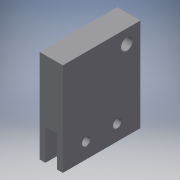
# Autodesk Inventor part: WideSupportForLift
Saved by Autodesk Inventor 2016 SP1 (Build 200210100, 210)
## iProperties
Created: 2016-02-14
Part Number: WideSupportForLift
Material: Aluminum 6061
Document SubType Name: Modeling
Designer: steele
Density: 2.7 g/cm^3
Appearance: Aluminum - Flat
Mass: 201.89 g
Surface Area: 182.87 cm^2
Volume: 74.7739 cm^3
Author: steele
Autodesk Inventor part; units mm, degrees
ref_plane "YZ Plane" through (0, 0, 0) normal (1, 0, 0) x (0, 1, 0)
ref_plane "XZ Plane" through (0, 0, 0) normal (0, 1, 0) x (-1, 0, 0)
ref_plane "XY Plane" through (0, 0, 0) normal (0, 0, 1) x (1, 0, 0)
sketch "Sketch6" plane through (0, 0, 0) normal (1, 0, 0) x (0, 1, 0)
  line L0 (-25.4, 31.75) -> (-25.4, -31.75)
  line L1 (-25.4, -31.75) -> (0, -31.75)
  line L2 (0, -31.75) -> (0, 31.75)
  line L3 (0, 31.75) -> (-25.4, 31.75)
  line L4 (-25.4, 31.75) -> (0, -31.75) construction
  line L5 (-25.4, -31.75) -> (0, 31.75) construction
  line L6 (0, 31.75) -> (0, -31.75)
  line L7 (0, -31.75) -> (50.8, -31.75)
  line L8 (50.8, -31.75) -> (50.8, 31.75)
  line L9 (50.8, 31.75) -> (0, 31.75)
  line L10 (0, 31.75) -> (50.8, -31.75) construction
  line L11 (0, -31.75) -> (50.8, 31.75) construction
  circle A0 centre (39.6875, -20.6375) radius 4.7625
  point P0 (0, 0)
  point P1 (-12.7, 0)
  point P2 (25.4, 0)
  dimension "d12" = 12.7
  dimension "d13" = 25.4
  dimension "d14" = 50.8
  dimension "d15" = 25.4
  dimension "d16" = 9.525
  dimension "d17" = 11.1125
  dimension "d18" = 11.1125
  dimension "d24" = 63.5
  constraints: 24 end point, 6 parallel, 4 midpoint, 2 perpendicular, 1 centre point, 1 vertical
  measures "d12" distance of point (-12.7, 0) point (0, 0)
  measures "d13" distance of point (0, 0) point (25.4, 0)
  measures "d14" distance of L8.end L6.start
  measures "d15" distance of L2.end L0.start
  measures "d16" diameter of A0
  measures "d17" distance from line of A0.centre L7
  measures "d18" distance from line of A0.centre L8
  measures "d24" distance of L0.start L0.end
extrude "Extrusion3" add sketch "Sketch6" along normal mid plane 19.05
sketch "Sketch7" plane through (-9.525, -25.4, 31.75) normal (0, 0, 1) x (1, 0, 0)
  line L0 (9.525, 25.4) -> (9.525, 0) construction
  line L1 (0, 0) -> (19.05, 0) construction
  line L2 (4.7625, 0) -> (14.2875, 0)
  line L3 (14.2875, 0) -> (14.2875, 25.4)
  line L4 (14.2875, 25.4) -> (4.7625, 25.4)
  line L5 (4.7625, 25.4) -> (4.7625, 0)
  line L6 (4.7625, 0) -> (14.2875, 25.4) construction
  line L7 (14.2875, 0) -> (4.7625, 25.4) construction
  point P0 (9.525, 12.7)
  dimension "d21" = 9.525
  constraints: 14 end point, 4 midpoint, 2 parallel, 1 horizontal, 1 perpendicular
  measures "d21" distance between parallel lines of L3 L5
extrude "Extrusion4" cut sketch "Sketch7" against normal through all
sketch "Sketch8" plane through (9.525, 0, 0) normal (1, 0, 0) x (0, 0, -1)
  line L0 (31.75, -25.4) -> (31.75, 0) projected
  line L1 (-31.75, -25.4) -> (31.75, -25.4) projected
  line L2 (-31.75, 0) -> (-31.75, -25.4) projected
  line L3 (-31.75, 0) -> (31.75, 0) projected
  line L4 (-292.1, -85.725) -> (-292.1, -12.7) projected
  arc A0 (-292.1, -85.725) -> (-279.4, -98.425) centre (-279.4, -85.725) ccw projected
  line L5 (222.25, -98.425) -> (-279.4, -98.425) projected
  arc A1 (222.25, -98.425) -> (234.95, -85.725) centre (222.25, -85.725) ccw projected
  line L6 (234.95, -81.1401) -> (234.95, -85.725) projected
  arc A2 (234.95, -81.1401) -> (231.6119, -72.5584) centre (222.25, -81.1401) ccw projected
  line L7 (231.6119, -72.5584) -> (168.8751, -4.1183) projected
  arc A3 (168.8751, -4.1183) -> (159.5132, 0) centre (159.5132, -12.7) ccw projected
  line L8 (159.5132, 0) -> (-279.4, 0) projected
  arc A4 (-279.4, 0) -> (-292.1, -12.7) centre (-279.4, -12.7) ccw projected
  circle A5 centre (215.9, -79.375) radius 4.826 projected
  circle A6 centre (-241.3, -79.375) radius 4.826 projected
  circle A7 centre (200.025, -79.375) radius 4.826 projected
  circle A8 centre (182.9995, -40.6685) radius 3.3782 projected
  circle A9 centre (165.1, -85.725) radius 3.3782 projected
  line L9 (-236.5375, -55.8157) -> (-236.5375, -25.4) projected
  arc A10 (-233.3625, -22.225) -> (-236.5375, -25.4) centre (-233.3625, -25.4) ccw projected
  line L10 (-233.3625, -22.225) -> (-210.2431, -22.225) projected
  arc A11 (-207.7154, -27.3213) -> (-210.2431, -22.225) centre (-210.2431, -25.4) ccw projected
  line L11 (-207.7154, -27.3213) -> (-230.8348, -57.737) projected
  arc A12 (-236.5375, -55.8157) -> (-230.8348, -57.737) centre (-233.3625, -55.8157) ccw projected
  line L12 (-229.0307, -71.1037) -> (-201.0846, -34.338) projected
  arc A13 (-195.3819, -36.2593) -> (-201.0846, -34.338) centre (-198.5569, -36.2593) ccw projected
  line L13 (-195.3819, -36.2593) -> (-195.3819, -73.025) projected
  arc A14 (-198.5569, -76.2) -> (-195.3819, -73.025) centre (-198.5569, -73.025) ccw projected
  line L14 (-198.5569, -76.2) -> (-226.503, -76.2) projected
  arc A15 (-229.0307, -71.1037) -> (-226.503, -76.2) centre (-226.503, -73.025) ccw projected
  line L15 (-73.119, -73.025) -> (-73.119, -34.8804) projected
  arc A16 (-67.6008, -32.738) -> (-73.119, -34.8804) centre (-69.944, -34.8804) ccw projected
  line L16 (-67.6008, -32.738) -> (-32.724, -70.8826) projected
  arc A17 (-35.0672, -76.2) -> (-32.724, -70.8826) centre (-35.0672, -73.025) ccw projected
  line L17 (-35.0672, -76.2) -> (-69.944, -76.2) projected
  arc A18 (-73.119, -73.025) -> (-69.944, -76.2) centre (-69.944, -73.025) ccw projected
  line L18 (34.0449, -27.5424) -> (-2.4193, -67.4233) projected
  arc A19 (-7.9375, -65.2808) -> (-2.4193, -67.4233) centre (-4.7625, -65.2808) ccw projected
  line L19 (-7.9375, -65.2808) -> (-7.9375, -25.4) projected
  arc A20 (-4.7625, -22.225) -> (-7.9375, -25.4) centre (-4.7625, -25.4) ccw projected
  line L20 (-4.7625, -22.225) -> (31.7017, -22.225) projected
  arc A21 (34.0449, -27.5424) -> (31.7017, -22.225) centre (31.7017, -25.4) ccw projected
  line L21 (-22.9807, -67.4233) -> (-59.4449, -27.5424) projected
  arc A22 (-57.1017, -22.225) -> (-59.4449, -27.5424) centre (-57.1017, -25.4) ccw projected
  line L22 (-57.1017, -22.225) -> (-20.6375, -22.225) projected
  arc A23 (-17.4625, -25.4) -> (-20.6375, -22.225) centre (-20.6375, -25.4) ccw projected
  line L23 (-17.4625, -25.4) -> (-17.4625, -65.2808) projected
  arc A24 (-22.9807, -67.4233) -> (-17.4625, -65.2808) centre (-20.6375, -65.2808) ccw projected
  line L24 (47.719, -34.8804) -> (47.719, -73.025) projected
  arc A25 (44.544, -76.2) -> (47.719, -73.025) centre (44.544, -73.025) ccw projected
  line L25 (44.544, -76.2) -> (9.6672, -76.2) projected
  arc A26 (7.324, -70.8826) -> (9.6672, -76.2) centre (9.6672, -73.025) ccw projected
  line L26 (7.324, -70.8826) -> (42.2008, -32.738) projected
  arc A27 (47.719, -34.8804) -> (42.2008, -32.738) centre (44.544, -34.8804) ccw projected
  line L27 (84.1375, -25.4) -> (84.1375, -73.025) projected
  arc A28 (80.9625, -76.2) -> (84.1375, -73.025) centre (80.9625, -73.025) ccw projected
  line L28 (80.9625, -76.2) -> (60.419, -76.2) projected
  arc A29 (57.244, -73.025) -> (60.419, -76.2) centre (60.419, -73.025) ccw projected
  line L29 (57.244, -73.025) -> (57.244, -25.4) projected
  arc A30 (60.419, -22.225) -> (57.244, -25.4) centre (60.419, -25.4) ccw projected
  line L30 (60.419, -22.225) -> (80.9625, -22.225) projected
  arc A31 (84.1375, -25.4) -> (80.9625, -22.225) centre (80.9625, -25.4) ccw projected
  line L31 (142.875, -69.85) -> (142.875, -29.1831) projected
  arc A32 (148.4044, -27.053) -> (142.875, -29.1831) centre (146.05, -29.1831) ccw projected
  line L32 (148.4044, -27.053) -> (188.0708, -70.8949) projected
  arc A33 (185.7165, -76.2) -> (188.0708, -70.8949) centre (185.7165, -73.025) ccw projected
  line L33 (185.7165, -76.2) -> (149.225, -76.2) projected
  arc A34 (142.875, -69.85) -> (149.225, -76.2) centre (149.225, -69.85) ccw projected
  circle A35 centre (-173.7792, -57.6072) radius 5.5626 projected
  circle A36 centre (-96.3092, -32.2072) radius 5.5626 projected
  circle A37 centre (-173.7792, -32.2072) radius 5.5626 projected
  circle A38 centre (-96.3092, -57.6072) radius 5.5626 projected
  circle A39 centre (101.6, -28.575) radius 2.5527 projected
  circle A40 centre (111.125, -19.05) radius 2.5527 projected
  circle A41 centre (120.65, -9.525) radius 2.5527 projected
  circle A42 centre (101.6, -88.9) radius 2.5527 projected
  circle A43 centre (120.65, -69.85) radius 2.5527 projected
  circle A44 centre (111.125, -79.375) radius 2.5527 projected
  circle A45 centre (-266.7, -12.7) radius 3.3782 projected
  circle A46 centre (-266.7, -85.725) radius 3.3782 projected
  circle A47 centre (-241.3, -12.7) radius 3.3782 projected
  circle A48 centre (-215.9, -12.7) radius 3.3782 projected
  circle A49 centre (-215.9, -85.725) radius 3.3782 projected
  circle A50 centre (-190.5, -12.7) radius 3.3782 projected
  circle A51 centre (-165.1, -12.7) radius 3.3782 projected
  circle A52 centre (-165.1, -85.725) radius 3.3782 projected
  circle A53 centre (-139.7, -12.7) radius 3.3782 projected
  circle A54 centre (-139.7, -85.725) radius 3.3782 projected
  circle A55 centre (-114.3, -12.7) radius 3.3782 projected
  circle A56 centre (-114.3, -85.725) radius 3.3782 projected
  circle A57 centre (-88.9, -12.7) radius 3.3782 projected
  circle A58 centre (-63.5, -12.7) radius 3.3782 projected
  circle A59 centre (-63.5, -85.725) radius 3.3782 projected
  circle A60 centre (-38.1, -12.7) radius 3.3782 projected
  circle A61 centre (-38.1, -85.725) radius 3.3782 projected
  circle A62 centre (-12.7, -12.7) radius 3.3782 projected
  circle A63 centre (12.7, -12.7) radius 3.3782 projected
  circle A64 centre (12.7, -85.725) radius 3.3782 projected
  circle A65 centre (38.1, -12.7) radius 3.3782 projected
  circle A66 centre (38.1, -85.725) radius 3.3782 projected
  circle A67 centre (63.5, -12.7) radius 3.3782 projected
  circle A68 centre (63.5, -85.725) radius 3.3782 projected
  circle A69 centre (88.9, -12.7) radius 3.3782 projected
  circle A70 centre (88.9, -85.725) radius 3.3782 projected
  circle A71 centre (139.7, -12.7) radius 3.3782 projected
  circle A72 centre (139.7, -85.725) radius 3.3782 projected
  circle A73 centre (161.925, -15.875) radius 4.953 projected
  circle A74 centre (-190.6194, -90.5002) radius 3.3528 projected
  circle A75 centre (-79.469, -90.5002) radius 3.3528 projected
  circle A76 centre (-135.0442, -60.325) radius 14.2812 projected
  circle A77 centre (-12.7, -83.185) radius 4.826 projected
  circle A78 centre (-12.7, -12.7) radius 3.3782
  circle A79 centre (12.7, -12.7) radius 3.3782
  point P0 (0, 0)
  constraints: 2 centre point, 2 coincident, 2 concentric
extrude "Extrusion5" cut sketch "Sketch8" against normal through all contours A62 | A63
body "Solid2"
